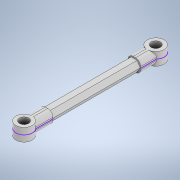
# Autodesk Inventor part: PX9200-19
Saved by Autodesk Inventor 2022.3 (Build 263350000, 350)
## iProperties
Created: 2022-07-14
Part Number: PX9200-19
Material: Generic
Document SubType Name: Modeling
Designer: luis_
Density: 1 g/cm^3
Appearance: Default
Author: luis_
Autodesk Inventor part; units mm, degrees
ref_plane "YZ Plane" through (0, 0, 0) normal (1, 0, 0) x (0, 1, 0)
ref_plane "XZ Plane" through (0, 0, 0) normal (0, 1, 0) x (-1, 0, 0)
ref_plane "XY Plane" through (0, 0, 0) normal (0, 0, 1) x (1, 0, 0)
sketch "Sketch1" plane through (0, 0, 0) normal (0, 0, 1) x (1, 0, 0)
  line L0 (2.3094, 0) -> (1.1547, -2)
  line L1 (1.1547, -2) -> (-1.1547, -2)
  line L2 (-1.1547, -2) -> (-2.3094, 0)
  line L3 (-2.3094, 0) -> (-1.1547, 2)
  line L4 (-1.1547, 2) -> (1.1547, 2)
  line L5 (1.1547, 2) -> (2.3094, 0)
  point P0 (0, 0)
  point P1 (0, 0)
  point P2 (0, -2)
  dimension "d0" = 4
  constraints: 12 end point, 1 coincident, 1 midpoint, 13 other
  measures "d0" distance from line of point (0, -2) L4
extrude "Extrusion1" add sketch "Sketch1" along normal blind 34.4
sketch "Sketch3" plane through (0, 0, 0) normal (0, 1, 0) x (-1, 0, 0)
  circle A0 centre (0.0059, -8.4136) radius 1.829
  line L0 (2.4692, 0) -> (2.4692, -6.2293)
  line L1 (-2.4692, -6.2426) -> (-2.4692, 0)
  arc A1 (-2.4692, -6.2426) -> (2.4692, -6.2293) centre (0.0059, -8.4136) ccw
  circle A2 centre (-0.0059, 43.2553) radius 1.829
  line L2 (-2.4692, 34.4) -> (-2.4692, 41.2059)
  line L3 (2.4692, 41.2201) -> (2.4692, 34.4)
  arc A3 (2.4692, 41.2201) -> (-2.4692, 41.2059) centre (-0.0059, 43.2553) ccw
  line L4 (1.1547, 34.4) -> (2.3094, 34.4) projected
  line L5 (2.4692, 34.4) -> (-2.4692, 34.4)
  line L6 (2.4692, 0) -> (-2.4692, 0)
  circle A4 centre (0.0059, -8.4136) radius 1.829
  point P0 (-1.1547, 34.4)
  constraints: 12 end point, 5 centre point, 4 point on circle, 3 coincident, 2 parallel, 1 concentric, 1 horizontal, 1 perpendicular
extrude "Extrusion3" add sketch "Sketch3" along normal mid plane 5 contours L2 A3 L3 L5 L4
extrude "Extrusion4" add sketch "Sketch3" along normal mid plane 5 contours L0 A1 L1 L6
fillet "Fillet1" radius 2 8 edges at (2.4692, 2.5, -3.1213) (-2.4692, 2.5, -3.1146) (2.4692, -2.5, -3.1213) (-2.4692, -2.5, -3.1146) (2.4692, -2.5, 37.803) (2.4692, 2.5, 37.803) (-2.4692, 2.5, 37.8101) (-2.4692, -2.5, 37.8101)
body "Solid1"
